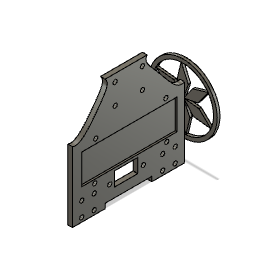
Simple_Robot_Body (Autodesk Fusion 360 design; units mm, degrees)
Autodesk Fusion 360 part; units mm, degrees
sketch "Sketch1" plane through (0, 0, 0) normal (1, 0, 0) x (0, 0, -1)
  line L0 (-50, 50) -> (70, 50)
  line L1 (70, 50) -> (70, -70)
  line L2 (70, -70) -> (-50, -70)
  line L3 (-50, -70) -> (-50, 50)
  circle A0 centre (-40, -50) radius 2.25
  circle A1 centre (-40.0426, -65.4999) radius 2.25
  circle A2 centre (-26.6, -50) radius 2.25
  circle A3 centre (-26.6, -65.4999) radius 2.25
  circle A4 centre (59.9574, -65.4999) radius 2.25
  circle A5 centre (46.5574, -65.4999) radius 2.25
  circle A6 centre (46.5574, -49.9999) radius 2.25
  circle A7 centre (59.9574, -49.9999) radius 2.25
  circle A8 centre (-10, -50) radius 2.25
  circle A9 centre (26, -50) radius 2.25
  line L4 (-40, -5) -> (62, -5)
  line L5 (62, -5) -> (62, -37.2)
  line L6 (62, -37.2) -> (-40, -37.2)
  line L7 (-40, -37.2) -> (-40, -5)
  line L8 (9.603, 32.6921) -> (9.603, 22.6921)
  circle A10 centre (-4.3722, 42.0822) radius 2.25
  circle A11 centre (24.8278, 42.0985) radius 2.25
  circle A12 centre (-4.2, 19.9828) radius 2.25
  circle A13 centre (25, 20) radius 2.25
  line L9 (-30, 5) -> (-20, 5)
  line L10 (-20, 5) -> (-20, -5)
  line L11 (-20, -5) -> (-30, -5)
  line L12 (-30, -5) -> (-30, 5)
  line L13 (45, 5) -> (55, 5)
  line L14 (55, 5) -> (55, -5)
  line L15 (55, -5) -> (45, -5)
  line L16 (45, -5) -> (45, 5)
  line L17 (-29.9622, -37.2) -> (-21.9622, -37.2)
  line L18 (-21.9622, -37.2) -> (-21.9622, -45.2)
  line L19 (-21.9622, -45.2) -> (-29.9622, -45.2)
  line L20 (-29.9622, -45.2) -> (-29.9622, -37.2)
  line L21 (55, -37.2) -> (47, -37.2)
  line L22 (47, -37.2) -> (47, -45.2)
  line L23 (47, -45.2) -> (55, -45.2)
  line L24 (55, -45.2) -> (55, -37.2)
  circle A14 centre (-25, 0) radius 2.25
  circle A15 centre (50, 0) radius 2.25
  circle A16 centre (51, -41) radius 2.25
  circle A17 centre (-26, -41) radius 2.25
  dimension "d1" = 120
  dimension "d2" = 120
  dimension "d3" = 4.5
  dimension "d4" = 4.5
  dimension "d5" = 15.5
  dimension "d6" = 4.5
  dimension "d7" = 13.4
  dimension "d8" = 4.5
  dimension "d9" = 4.5
  dimension "d10" = 100
  dimension "d11" = 4.5
  dimension "d12" = 13.4
  dimension "d13" = 4.5
  dimension "d14" = 15.5
  dimension "d15" = 4.5
  dimension "d16" = 4.5
  dimension "d17" = 4.5
  dimension "d18" = 36
  dimension "d19" = 32.2
  dimension "d20" = 102
  dimension "d21" = 4.5
  dimension "d22" = 4.5
  dimension "d23" = 29.2
  dimension "d24" = 4.5
  dimension "d25" = 4.5
  dimension "d26" = 29.2
  dimension "d27" = 22.1
  dimension "d28" = 10
  dimension "d29" = 10
  dimension "d30" = 10
  dimension "d31" = 10
  dimension "d32" = 8
  dimension "d33" = 8
  dimension "d34" = 8
  dimension "d35" = 8
  dimension "d38" = 4.5
  dimension "d39" = 4.5
  dimension "d40" = 4.5
  dimension "d41" = 4.5
  constraint horizontal L0
  constraint vertical L1
  constraint horizontal L2
  constraint vertical L3
  constraint horizontal L4
  constraint vertical L5
  constraint horizontal L6
  constraint vertical L7
  constraint vertical L8
  constraint horizontal L9
  constraint vertical L10
  constraint horizontal L11
  constraint vertical L12
  constraint horizontal L13
  constraint vertical L14
  constraint horizontal L15
  constraint vertical L16
  constraint horizontal L17
  constraint vertical L18
  constraint horizontal L19
  constraint vertical L20
  constraint coincident L6 L17.start
  constraint horizontal L21
  constraint vertical L22
  constraint horizontal L23
  constraint vertical L24
  constraint coincident L6 L21.start
  measures "d1" distance of L0.start L0.end
  measures "d2" distance of L0.start L2.end
  measures "d3" diameter of A0
  measures "d4" diameter of A1
  measures "d5" distance of A0.centre A1.centre
  measures "d6" diameter of A2
  measures "d7" distance of A0.centre A2.centre
  measures "d8" diameter of A3
  measures "d9" diameter of A4
  measures "d10" distance of A1.centre A4.centre
  measures "d11" diameter of A5
  measures "d12" distance of A4.centre A5.centre
  measures "d13" diameter of A6
  measures "d14" distance of A5.centre A6.centre
  measures "d15" diameter of A7
  measures "d16" diameter of A8
  measures "d17" diameter of A9
  measures "d18" distance of A8.centre A9.centre
  measures "d19" distance of L4.start L6.end
  measures "d20" distance of L4.start L4.end
  measures "d21" diameter of A10
  measures "d22" diameter of A11
  measures "d23" distance of A10.centre A11.centre
  measures "d24" diameter of A12
  measures "d25" diameter of A13
  measures "d26" distance of A12.centre A13.centre
  measures "d27" distance of A10.centre A12.centre
  measures "d28" distance of L9.start L9.end
  measures "d29" distance of L9.start L11.end
  measures "d30" distance of L13.start L13.end
  measures "d31" distance of L13.start L15.end
  measures "d32" distance of L17.start L17.end L0.start
  measures "d33" distance of L17.start L19.end
  measures "d34" distance of L21.start L23.end
  measures "d35" distance of L21.start L21.end L0.start
  measures "d38" diameter of A14
  measures "d39" diameter of A15
  measures "d40" diameter of A16
  measures "d41" diameter of A17
extrude "Extrude2" add sketch "Sketch1" along normal blind 5 contours L4 L9 L10 L11 L12 | L6 L17 L18 L19 L20 | L4 L13 L14 L15 L16 | L6 L21 L22 L23 L24 makes body 1 at (0, -4.0812, -50.056) makes body 2 at (3.3333, -41.224, -48.7612) makes body 3 at (0, -4.0812, 24.944) makes body 4 at (3.3333, -41.224, 28.2388)
extrude "Extrude1" add sketch "Sketch1" along normal blind 5 separate body contours L0 L1 L2 L3 makes body 5
extrude "Extrude3" add sketch "Sketch1" along normal blind 3 contours L4 L5 L6 L7 L11 L15 L17 L21 bodies 1 2 3 4 5
sketch "Sketch2" plane through (5, 0, 0) normal (1, 0, 0) x (0, 0, -1)
  circle A0 centre (50, 0) radius 2.25
  circle A1 centre (51, -41) radius 2.25
  circle A2 centre (25, 20) radius 2.25
  circle A3 centre (-4.2, 19.9828) radius 2.25
  circle A4 centre (24.8278, 42.0985) radius 2.25
  circle A5 centre (-4.3722, 42.0822) radius 2.25
  circle A6 centre (26, -50) radius 2.25
  circle A7 centre (-10, -50) radius 2.25
  circle A8 centre (59.9574, -49.9999) radius 2.25
  circle A9 centre (46.5574, -49.9999) radius 2.25
  circle A10 centre (59.9574, -65.4999) radius 2.25
  circle A11 centre (-26.6, -65.4999) radius 2.25
  circle A12 centre (-26.6, -50) radius 2.25
  circle A13 centre (-40.0426, -65.4999) radius 2.25
  circle A14 centre (-40, -50) radius 2.25
  circle A15 centre (46.5574, -65.4999) radius 2.25
  line L0 (-50, -70) -> (70, -70)
  line L1 (70, -70) -> (70, 50)
  line L2 (70, 50) -> (-50, 50)
  line L3 (-50, 50) -> (-50, -70)
  circle A16 centre (-26, -41) radius 2.25
  circle A17 centre (-25, 0) radius 2.25
  line L4 (-40, -5) -> (62, -5)
  line L5 (62, -5) -> (62, -37.2)
  line L6 (62, -37.2) -> (-40, -37.2)
  line L7 (-40, -37.2) -> (-40, -5)
  line L8 (-5, -40) -> (20, -40)
  line L9 (20, -40) -> (20, -55)
  line L10 (20, -55) -> (-5, -55)
  line L11 (-5, -55) -> (-5, -40)
  constraint horizontal L8
  constraint vertical L9
  constraint horizontal L10
  constraint vertical L11
extrude "Extrude5" cut sketch "Sketch2" against normal blind 5 contours L8 L9 L10 L11 bodies 1
sketch "Sketch3" plane through (5, 0, 0) normal (1, 0, 0) x (0, 0, -1)
  circle A0 centre (50, 0) radius 2.25
  circle A1 centre (51, -41) radius 2.25
  circle A2 centre (25, 20) radius 2.25
  circle A3 centre (-4.2, 19.9828) radius 2.25
  circle A4 centre (24.8278, 42.0985) radius 2.25
  circle A5 centre (-4.3722, 42.0822) radius 2.25
  circle A6 centre (26, -50) radius 2.25
  circle A7 centre (-10, -50) radius 2.25
  circle A8 centre (59.9574, -49.9999) radius 2.25
  circle A9 centre (46.5574, -49.9999) radius 2.25
  circle A10 centre (59.9574, -65.4999) radius 2.25
  circle A11 centre (-26.6, -65.4999) radius 2.25
  circle A12 centre (-26.6, -50) radius 2.25
  circle A13 centre (-40.0426, -65.4999) radius 2.25
  circle A14 centre (-40, -50) radius 2.25
  circle A15 centre (46.5574, -65.4999) radius 2.25
  line L0 (-50, -70) -> (70, -70)
  line L1 (70, -70) -> (70, 50)
  line L2 (70, 50) -> (-50, 50)
  line L3 (-50, 50) -> (-50, -70)
  circle A16 centre (-26, -41) radius 2.25
  circle A17 centre (-25, 0) radius 2.25
  line L4 (-40, -5) -> (62, -5)
  line L5 (62, -5) -> (62, -37.2)
  line L6 (62, -37.2) -> (-40, -37.2)
  line L7 (-40, -37.2) -> (-40, -5)
  spline S0 degree 5 poles (-15, 50) (-14.3034, 49.2482) (-13.1782, 47.6882) (-12.3216, 45.1976) (-12.8241, 41.5409) (-15.7347, 36.0901) (-20.2606, 29.52) (-25.7387, 22.0091) (-31.6928, 14.4328) (-37.7621, 8.0159) (-43.6521, 4.0483) (-49.0747, 3.5639) (-53.7012, 7.0619) (-57.0907, 14.1181) (-58.7593, 23.5815) (-58.2881, 33.9264) (-55.422, 43.5432) (-50.1744, 51.0472) (-42.9414, 55.5903) (-34.6058, 57.1567) (-26.3033, 56.2572) (-20.6265, 54.1805) (-17.3578, 52.1988) (-15.6966, 50.7518) (-15, 50) knots 0 0 0 0 0 0 0.05 0.1 0.15 0.2 0.25 0.3 0.35 0.4 0.45 0.5 0.55 0.6 0.65 0.7 0.75 0.8 0.85 0.9 0.95 1 1 1 1 1 1
  spline S1 degree 5 poles (30, 50) (29.4137, 49.2485) (28.5748, 47.7025) (28.3336, 45.2707) (29.9376, 41.7429) (34.3463, 36.4511) (40.1385, 29.9583) (46.4026, 22.3907) (52.6397, 14.655) (58.6158, 8.0682) (64.2367, 4.0257) (69.4121, 3.6448) (73.9375, 7.4403) (77.3379, 14.9035) (78.995, 24.7697) (78.3191, 35.3905) (74.9131, 45.0692) (68.7293, 52.3846) (60.2762, 56.5779) (50.691, 57.7538) (41.3939, 56.5125) (35.3367, 54.2578) (32.0926, 52.2118) (30.5863, 50.7515) (30, 50) knots 0 0 0 0 0 0 0.05 0.1 0.15 0.2 0.25 0.3 0.35 0.4 0.45 0.5 0.55 0.6 0.65 0.7 0.75 0.8 0.85 0.9 0.95 1 1 1 1 1 1
  line L8 (20, -40) -> (20, -55)
  line L9 (20, -55) -> (-5, -55)
  line L10 (-5, -55) -> (-5, -40)
  line L11 (-5, -40) -> (20, -40)
  point P0 (-20, 30)
  point P1 (-50, 5)
  point P2 (-50, 50)
  point P3 (40, 30)
  point P4 (70, 5)
  point P5 (70, 50)
  constraint coincident L2 S0.start
  constraint coincident L3 P1
  constraint coincident P2 L2.end
  constraint coincident L2 S1.start
  constraint coincident L1 P4
  constraint coincident P5 L1.end
extrude "Extrude4" cut sketch "Sketch3" against normal blind 5 contours L2 L3 S0 | L1 L2 S1 bodies 1
sketch "Sketch4" plane through (5, 0, 0) normal (1, 0, 0) x (0, 0, -1)
  line L0 (-40, -5) -> (62, -5)
  line L1 (62, -5) -> (62, -37.2)
  line L2 (62, -37.2) -> (-40, -37.2)
  line L3 (-40, -37.2) -> (-40, -5)
  circle A0 centre (-25, 0) radius 2.25
  circle A1 centre (-26, -41) radius 2.25
  spline S0 degree 5 poles (-15, 50) (-14.3034, 49.2482) (-13.1782, 47.6882) (-12.3216, 45.1976) (-12.8241, 41.5409) (-15.7347, 36.0901) (-20.2606, 29.52) (-25.7387, 22.0091) (-31.6928, 14.4328) (-37.7621, 8.0159) (-42.7449, 4.6594) (-46.3059, 3.9133) (-48.5874, 4.3564) (-49.7796, 4.8902) (-50, 5) knots 0 0 0 0 0 0 0.05 0.1 0.15 0.2 0.25 0.3 0.35 0.4 0.45 0.461493 0.461493 0.461493 0.461493 0.461493 0.461493
  line L4 (-50, 5) -> (-50, -70)
  line L5 (-50, -70) -> (70, -70)
  line L6 (70, -70) -> (70, 5)
  spline S1 degree 5 poles (70, 5) (69.8513, 4.9261) (68.7541, 4.4208) (66.618, 3.9791) (63.29, 4.7065) (58.6158, 8.0682) (52.6397, 14.655) (46.4026, 22.3907) (40.1385, 29.9583) (34.3463, 36.4511) (29.9376, 41.7429) (28.3336, 45.2707) (28.5748, 47.7025) (29.4137, 49.2485) (30, 50) knots -0.457897 -0.457897 -0.457897 -0.457897 -0.457897 -0.457897 -0.45 -0.4 -0.35 -0.3 -0.25 -0.2 -0.15 -0.1 -0.05 0 0 0 0 0 0
  line L7 (30, 50) -> (-15, 50)
  circle A2 centre (46.5574, -65.4999) radius 2.25
  circle A3 centre (-40, -50) radius 2.25
  circle A4 centre (-40.0426, -65.4999) radius 2.25
  circle A5 centre (-26.6, -50) radius 2.25
  circle A6 centre (-26.6, -65.4999) radius 2.25
  circle A7 centre (59.9574, -65.4999) radius 2.25
  circle A8 centre (46.5574, -49.9999) radius 2.25
  circle A9 centre (59.9574, -49.9999) radius 2.25
  circle A10 centre (-10, -50) radius 2.25
  circle A11 centre (26, -50) radius 2.25
  circle A12 centre (-4.3722, 42.0822) radius 2.25
  circle A13 centre (24.8278, 42.0985) radius 2.25
  circle A14 centre (-4.2, 19.9828) radius 2.25
  circle A15 centre (25, 20) radius 2.25
  circle A16 centre (51, -41) radius 2.25
  circle A17 centre (50, 0) radius 2.25
  line L8 (20, -40) -> (20, -55)
  line L9 (20, -55) -> (-5, -55)
  line L10 (-5, -55) -> (-5, -40)
  line L11 (-5, -40) -> (20, -40)
  line L12 (-14.9357, -65) -> (35, -65)
  line L13 (35, -65) -> (35, -70)
  line L14 (35, -70) -> (-14.9357, -70)
  line L15 (-14.9357, -70) -> (-14.9357, -65)
  constraint horizontal L12
  constraint vertical L13
  constraint horizontal L14
  constraint vertical L15
  constraint coincident L5 L13.end
extrude "Extrude6" cut sketch "Sketch4" against normal blind 5 contours L5 L12 L13 L14 L15 bodies 1
sketch "Sketch5" plane through (0, 0, 0) normal (0, 0, 1) x (1, 0, 0)
  circle A0 centre (-60, 0) radius 32.5
  circle A1 centre (-60, 0) radius 36.4005
  line L0 (-60, 0) -> (-65, -15)
  line L1 (-65, -15) -> (-57.4067, -32.3964)
  line L2 (-60, 0) -> (-53.2461, -15)
  line L3 (-53.2461, -15) -> (-57.4067, -32.3964)
  dimension "d52" = 65
  constraint concentric A0 A1
  constraint coincident A0.centre A1.centre
  constraint coincident A0 L1.end
  measures "d52" diameter of A0
extrude "Extrude7" add sketch "Sketch5" along normal blind 3 separate body contours A1 makes body 6
extrude "Extrude8" add sketch "Sketch5" along normal blind 2.5 separate body contours L0 L1 L2 L3 makes body 7
pattern_circular "C-Pattern1" count 6 over 360 about axis through (-60, 0, 0) along (0, 0, 1) of bodies 7 makes body 8 at (-41.2632, -9.1445, 0) makes body 9 at (-42.7123, 11.6543, 0) makes body 10 at (-61.4491, 20.7988, 0) makes body 11 at (-78.7368, 9.1445, 0) makes body 12 at (-77.2877, -11.6543, 0)
move_body "Move1" bodies 1 to x (1, 0, 0) y (0, 1, 0) z (0, 0, 1) at (-2.4705, 11.9626, 10)
move_body "Move2" bodies 11 9 10 8 6 7 12 to x (1, 0, 0) y (0, 1, 0) z (0, 0, 1) at (60, 0, 0)
move_body "Move3" bodies 12 9 10 11 8 7 6 to x (1, 0, 0) y (0, 1, 0) z (0, 0, 1) at (0, 0, -64)
